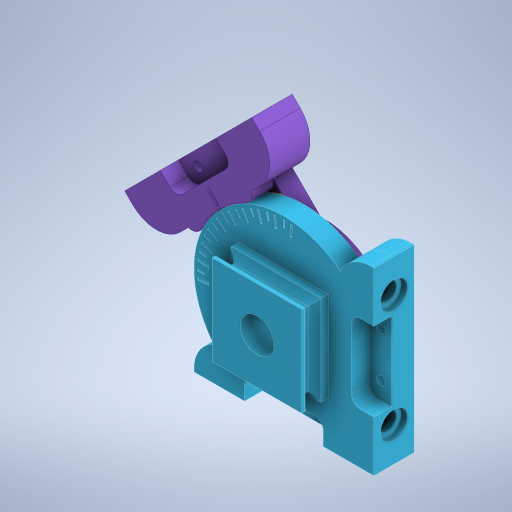
# Autodesk Inventor part: Rail-AdjustableAngle
Saved by Autodesk Inventor 2023.1 (Build 271208000, 208)
## iProperties
Created: 2023-06-07
Part Number: Rail-AdjustableAngle
Material: ABS Plastic
Document SubType Name: Modeling
Designer: hello
Density: 1.06 g/cm^3
Appearance: Turquoise
Author: hello
Autodesk Inventor part; units mm, degrees
ref_plane "YZ Plane" through (0, 0, 0) normal (1, 0, 0) x (0, 1, 0)
ref_plane "XZ Plane" through (0, 0, 0) normal (0, 1, 0) x (-1, 0, 0)
ref_plane "XY Plane" through (0, 0, 0) normal (0, 0, 1) x (1, 0, 0)
sketch "Sketch1" plane through (0, 0, 0) normal (0, 0, 1) x (1, 0, 0)
  line L0 (-40, 40) -> (40, 40)
  line L1 (40, 40) -> (40, -40)
  line L2 (40, -40) -> (-40, -40)
  line L3 (-40, -40) -> (-40, 40)
  line L4 (-40, 40) -> (40, -40) construction
  line L5 (40, 40) -> (-40, -40) construction
  line L6 (40, 0) -> (-40, 0) construction
  arc A0 (0, 40) -> (-39.8798, -3.0986) centre (0, 0) ccw
  point P0 (0, 0)
  point P1 (-40, -18.9335)
  point P2 (0, 0)
  point P3 (-40, 0)
  dimension "d0" = 80
  dimension "d1" = 80
  constraints: 14 end point, 6 midpoint, 2 horizontal, 2 parallel, 2 point on circle, 1 centre point, 1 coincident, 1 perpendicular, 1 point on line
  measures "d0" distance of L1.end L2.end
  measures "d1" distance of L0.end L1.end
extrude "Extrusion1" add sketch "Sketch1" along normal blind 18 contours L0 L1 L2 L3 A0
sketch "Sketch2" plane through (40, -40, 0) normal (1, 0, 0) x (0, 0, -1)
  line L0 (0, 0) -> (0, 80) projected
  line L1 (0, 80) -> (-18, 80) projected
  line L2 (-18, 0) -> (-18, 80) projected
  line L3 (0, 0) -> (-18, 0) projected
  line L4 (-9, 15) -> (-9, 65)
  point P0 (0, 40)
  point P1 (-9, 40)
  point P2 (0, 40)
  point P3 (-9, 0)
  dimension "d7" = 50
  constraints: 3 midpoint, 2 coincident, 2 end point, 1 horizontal alignment, 1 vertical, 1 vertical alignment
  measures "d7" distance of L4.start L4.end
hole "Hole1" at (40, -25, 9) at (40, 25, 9) direction (-1, 0, 0) diameter 8.05 depth 15 counterbore diameter 12 counterbore depth 3
sketch "Sketch3" plane through (-40, -40, 0) normal (0, -1, 0) x (1, 0, 0)
  line L0 (0, 0) -> (80, 0) projected
  line L1 (80, 0) -> (80, 18) projected
  line L2 (0, 18) -> (80, 18) projected
  line L3 (0, 0) -> (0, 18) projected
  line L4 (15, 9) -> (65, 9)
  point P0 (40, 0)
  point P1 (40, 9)
  point P2 (0, 9)
  point P3 (40, 0)
  dimension "d15" = 50
  constraints: 3 midpoint, 2 coincident, 2 end point, 1 horizontal, 1 horizontal alignment, 1 vertical alignment
  measures "d15" distance of L4.start L4.end
hole "Hole2" at (-25, -40, 9) at (25, -40, 9) direction (0, 1, 0) diameter 8.05 depth 15 counterbore diameter 12 counterbore depth 3
sketch "Sketch4" plane through (0, 0, 18) normal (0, 0, 1) x (1, 0, 0)
  line L0 (40, -40) -> (40, 40) projected
  line L1 (34, -17.5) -> (40, -17.5)
  line L2 (40, -17.5) -> (40, 17.5)
  line L3 (40, 17.5) -> (34, 17.5)
  line L4 (30, 13.5) -> (30, -13.5)
  arc A0 (30, -13.5) -> (34, -17.5) centre (34, -13.5) ccw
  arc A1 (34, 17.5) -> (30, 13.5) centre (34, 13.5) ccw
  point P0 (0, 0)
  point P1 (30, -17.5)
  point P2 (30, 17.5)
  point P3 (40, 0)
  dimension "d23" = 35
  dimension "d24" = 10
  dimension "d25" = 4
  constraints: 8 end point, 4 point on circle, 4 point on line, 4 tangent, 2 centre point, 2 midpoint, 2 parallel, 1 equal radius, 1 horizontal, 1 perpendicular
  measures "d23" distance of point (30, 17.5) point (30, -17.5)
  measures "d24" distance of point (30, -17.5) L1.end
  measures "d25" radius of A0
extrude "Extrusion2" cut sketch "Sketch4" against normal blind 8
sketch "Sketch5" plane through (0, 0, 10) normal (0, 0, 1) x (1, 0, 0)
  line L0 (35, -10) -> (35, 10)
  line L1 (40, 17.5) -> (40, -17.5) projected
  point P0 (0, 0)
  point P1 (35, 0)
  point P2 (40, 0)
  dimension "d28" = 20
  dimension "d29" = 5
  constraints: 2 coincident, 2 end point, 2 midpoint, 1 horizontal alignment, 1 vertical
  measures "d28" distance of L0.start L0.end
  measures "d29" distance between parallel lines of L1 L0
hole "Hole3" at (35, -10, 10) at (35, 10, 10) direction (0, 0, -1) diameter 4 depth 5
pattern_circular "Circular Pattern1" count 2 over 90 about axis through (0, 0, -10) along (0, 0, -1) of "Extrusion2", "Hole3"
sketch "Sketch6" plane through (0, 0, 18) normal (0, 0, 1) x (1, 0, 0)
  line L0 (-20, 20) -> (20, 20)
  line L1 (20, 20) -> (20, -20)
  line L2 (20, -20) -> (-20, -20)
  line L3 (-20, -20) -> (-20, 20)
  line L4 (-20, 20) -> (20, -20) construction
  line L5 (20, 20) -> (-20, -20) construction
  point P0 (0, 0)
  dimension "d40" = 40
  dimension "d41" = 40
  constraints: 12 end point, 2 midpoint, 2 parallel, 1 horizontal, 1 perpendicular
  measures "d40" distance of L1.end L2.end
  measures "d41" distance of L0.end L1.end
extrude "Extrusion3" add sketch "Sketch6" along normal blind 12
sketch "Sketch11" plane through (-20, -20, 18) normal (0, -1, 0) x (1, 0, 0)
  line L0 (40, 0) -> (0, 0) projected
  line L1 (40, 0) -> (40, 12) projected
  line L2 (0, 12) -> (40, 12) construction
  line L3 (0, 0) -> (0, 12) construction
  line L4 (0, 12) -> (40, 12) projected
  line L5 (0, 12) -> (0, 10)
  line L6 (0, 0) -> (0, 12) projected
  circle A0 centre (0, 6.7947) radius 3 construction
  arc A1 (4.3, 6.7947) -> (0, 10) centre (-2.036, 2.7817) ccw
  arc A2 (0, 3.5894) -> (4.3, 6.7947) centre (-2.036, 10.8077) ccw
  line L7 (3.5, 7.8415) -> (3.5, 5.7479)
  line L8 (0, 10) -> (0, 3.5894)
  point P0 (20, -18)
  point P1 (0, 11)
  dimension "d65" = 2
  dimension "d66" = 6
  dimension "d67" = 7.5
  dimension "d68" = 7.5
  dimension "d69" = 3.5
  dimension "d70" = 4.3
  constraints: 6 end point, 6 point on circle, 3 centre point, 3 point on line, 2 tangent, 2 vertical, 1 horizontal alignment, 1 midpoint
  measures "d65" distance of L2.start L5.end
  measures "d66" diameter of A0
  measures "d67" radius of A1
  measures "d68" radius of A2
  measures "d69" distance from line of L7 point (0, 11)
  measures "d70" distance from line of A1.start L3
extrude "Extrusion5" cut sketch "Sketch11" against normal through all contours L6 A1 L7 A2
pattern_circular "Circular Pattern2" count 4 over 360 about axis through (0, 0, -10) along (0, 0, 1) of "Extrusion5"
fillet "Fillet1" radius 1.5 4 edges at (0, -20, 28) (-20, 0, 28) (0, 20, 28) (20, 0, 28)
sketch "Sketch12" plane through (0, 0, 30) normal (0, 0, 1) x (1, 0, 0)
  point P0 (0, 0)
  point P1 (0, 0)
  constraints: 1 coincident
hole "Hole6" at (0, 0, 30) direction (0, 0, -1) diameter 5.5 end through all counterbore diameter 15 counterbore depth 20 clearance for "Hex Head Cap Screw ISO 24017" size "M5" standard "ISO"
sketch "Sketch17" plane through (0, 0, 0) normal (0, 0, -1) x (-1, 0, 0)
  arc A0 (40, 0) -> (0, 40) centre (0, 0) ccw projected
  arc A1 (31.225, -25) -> (40, 0) centre (0, 0) ccw
  line L0 (40, 0) -> (40, -40) projected
  line L1 (40, 0) -> (40, -25)
  line L2 (31.225, -25) -> (40, -25)
  line L3 (-40, 40) -> (0, 40) projected
  arc A2 (0, 40) -> (-25, 31.225) centre (0, 0) ccw
  line L4 (-25, 31.225) -> (-25, 40)
  line L5 (-25, 40) -> (0, 40)
  point P0 (0, 0)
  dimension "d118" = 40
  dimension "d119" = 25
  dimension "d122" = 40
  dimension "d123" = 25
  constraints: 8 end point, 4 point on circle, 3 perpendicular, 3 tangent, 2 centre point, 2 point on line
  measures "d118" radius of A1
  measures "d119" vertical distance of L2.start point (0, 0)
  measures "d122" radius of A2
  measures "d123" horizontal distance of point (0, 0) L4.start
extrude "Extrusion8" cut sketch "Sketch17" against normal through all
sketch "Sketch18" plane through (0, 0, 0) normal (0, 0, -1) x (-1, 0, 0)
  arc A0 (31.225, -25) -> (-25, 31.225) centre (0, 0) ccw projected
  arc A1 (31.225, -25) -> (-25, 31.225) centre (0, 0) ccw projected
  line L0 (-25, 31.225) -> (31.225, -25)
  circle A2 centre (0, 0) radius 2.75 projected
  circle A3 centre (0, 0) radius 30
  point P0 (24.0961, -17.8711)
  point P1 (-17.8711, 24.0961)
  dimension "d124" = 60
  constraints: 2 end point, 1 centre point, 1 coincident
  measures "d124" diameter of A3
extrude "Extrusion9" cut sketch "Sketch18" against normal blind 9
sketch "Sketch19" plane through (0, 0, 0) normal (0, 1, 0) x (-1, 0, 0)
  line L0 (-2.75, 9) -> (2.75, 9) projected
  line L1 (2.75, 9) -> (2.75, 0)
  line L2 (2.75, 9) -> (25, 9)
  line L3 (24.0961, 9) -> (-30, 9) projected
  line L4 (25, 9) -> (25, 0)
  line L5 (40, 0) -> (-40, 0) projected
  line L6 (2.75, 0) -> (25, 0)
  line L7 (0, 0) -> (0, 9)
  circle A0 centre (25, 4.5) radius 3
  point P0 (-17.8711, 9)
  point P1 (25, 1.5)
  point P2 (25, 7.5)
  dimension "d128" = 50
  dimension "d129" = 6
  constraints: 10 end point, 3 point on line, 2 perpendicular, 1 centre point, 1 collinear, 1 midpoint, 1 vertical
  measures "d128" diameter of L4 L7
  measures "d129" diameter of A0
revolve "Revolution1" add sketch "Sketch19" angle 360 about axis through (0, 0, 0) along (0, 0, 1) contours L2 L4 A0 L5 L1
fillet "Fillet3" radius 15 2 edges at (17.8711, 24.0961, 4.5) (-24.0961, -17.8711, 4.5)
fillet "Fillet4" radius 15 2 edges at (25, 40, 9) (-40, -25, 9)
sketch "Sketch20" plane through (0, 0, 0) normal (0, 1, 0) x (-1, 0, 0)
  arc A0 (25, 7.5) -> (25, 1.5) centre (25, 4.5) ccw projected
  line L0 (25, 7.5) -> (25, 9) projected
  line L1 (25, 0) -> (25, 1.5) projected
  arc A1 (25.1, 7.2982) -> (25.1, 1.7018) centre (25, 4.5) ccw
  line L2 (25.1, 7.2982) -> (25.1, 9)
  line L3 (25.1, 0) -> (25.1, 1.7018)
  line L4 (25.1, 0) -> (29.9, 0)
  line L5 (40, 0) -> (-40, 0) projected
  line L6 (29.9, 0) -> (29.9, 8.6)
  line L7 (29.9, 8.6) -> (25.1, 8.6)
  line L8 (0, -6) -> (0, 36) projected
  point P0 (0, 0)
  dimension "d133" = 0.2
  dimension "d134" = 0.1
  dimension "d135" = 0.1
  dimension "d136" = 0.4
  dimension "d137" = 4.9
  constraints: 10 end point, 2 parallel, 2 point on circle, 2 point on line, 1 centre point, 1 horizontal, 1 horizontal alignment, 1 vertical
  measures "d133" radial gap between concentric circles of A0 A1
  measures "d134" distance between parallel lines of L0 L2
  measures "d135" distance between parallel lines of L1 L3
  measures "d136" distance from line of L2.end L7
  measures "d137" distance from line of L6 A0.centre
revolve "Revolution2" add sketch "Sketch20" angle 360 about axis through (0, 0, -10) along (0, 0, 1) separate body
sketch "Sketch21" plane through (0, 0, 0) normal (0, 0, -1) x (-1, 0, 0)
  circle A0 centre (0, 0) radius 29.9 projected
  circle A1 centre (0, 0) radius 29.9 projected
  line L0 (1.5743, 29.8585) -> (14.3022, 42.5865)
  line L1 (14.3022, 42.5865) -> (42.5865, 14.3022)
  line L2 (42.5865, 14.3022) -> (29.8585, 1.5743)
  circle A2 centre (0, 0) radius 2.75 projected
  line L3 (0, 0) -> (28.4443, 28.4443)
  line L4 (0, 0) -> (0, 11.9435)
  line L5 (14.3022, 42.5865) -> (0.16, 56.7286)
  line L6 (0.16, 56.7286) -> (14.3022, 70.8707)
  line L7 (14.3022, 70.8707) -> (70.8707, 14.3022)
  line L8 (70.8707, 14.3022) -> (56.7286, 0.16)
  line L9 (56.7286, 0.16) -> (42.5865, 14.3022)
  point P0 (29.8585, 1.5743)
  dimension "d139" = 40
  dimension "d140" = 18
  dimension "d141" = 45
  dimension "d142" = 20
  dimension "d143" = 80
  constraints: 20 end point, 7 perpendicular, 2 collinear, 2 point on circle, 1 midpoint, 1 vertical
  measures "d139" distance of L0.end L1.end
  measures "d140" distance of L1.end L2.end
  measures "d141" angle of L3 L4
  measures "d142" distance of L7.end L8.end
  measures "d143" distance of L6.end L7.end
extrude "Extrusion10" add sketch "Sketch21" against normal up to surface (8.6 mm away) contours A0 L3 L1 L2 | L0 L1 L3 A0 | L1 L5 L6 L7 L8 L9 bodies 2
sketch "Sketch22" plane through (0, 0, 8.6) normal (0, 0, 1) x (0.7071068, -0.7071068, 0)
  circle A0 centre (0, 0) radius 25.1 projected
  arc A1 (-22.2263, -20) -> (-22.2263, 20) centre (0, 0) ccw projected
  line L0 (-40.2263, 20) -> (-22.2263, 20) projected
  line L1 (-40.2263, 40) -> (-40.2263, 20) projected
  line L2 (-60.2263, 40) -> (-40.2263, 40) projected
  line L3 (-60.2263, -40) -> (-60.2263, 40) projected
  line L4 (-40.2263, -40) -> (-60.2263, -40) projected
  line L5 (-40.2263, -20) -> (-40.2263, -40) projected
  line L6 (-22.2263, -20) -> (-40.2263, -20) projected
  circle A2 centre (0, 0) radius 2.75 projected
  circle A3 centre (0, 0) radius 40.25
  point P0 (-34.9294, -20)
  point P1 (-34.9294, 20)
  dimension "d146" = 80.5
  constraints: 1 centre point, 1 coincident
  measures "d146" diameter of A3
extrude "Extrusion11" add sketch "Sketch22" along normal up to surface (9.4 mm away) contours L6 L5 L4 L3 L2 L1 L0 A3 bodies 2
sketch "Sketch23" plane through (-14.3022, 70.8707, 0) normal (-0.7071068, 0.7071068, 0) x (-0.7071068, -0.7071068, 0)
  line L0 (0, 0) -> (0, 18) projected
  line L1 (80, 0) -> (0, 0) projected
  line L2 (80, 0) -> (80, 18) projected
  line L3 (80, 18) -> (0, 18) projected
  line L4 (15, 9) -> (65, 9)
  line L5 (80, 0) -> (0, 0) projected
  point P0 (40, 0)
  point P1 (40, 9)
  point P2 (0, 9)
  point P3 (40, 0)
  dimension "d149" = 50
  constraints: 3 midpoint, 2 coincident, 2 end point, 1 horizontal, 1 horizontal alignment, 1 vertical alignment
  measures "d149" distance of L4.start L4.end
hole "Hole7" at (-24.9088, 60.2641, 9) at (-60.2641, 24.9088, 9) direction (0.7071068, -0.7071068, 0) diameter 8.05 depth 15 counterbore diameter 12 counterbore depth 3 bodies 2
fillet "Fillet5" radius 5 2 edges at (-10.5567, 38.8409, 13.3) (-38.8409, 10.5567, 13.3)
sketch "Sketch24" plane through (0, 0, 0) normal (0, 1, 0) x (-1, 0, 0)
  line L0 (36.5062, 8.6) -> (16.9516, 8.6) construction
  line L1 (40, 9) -> (-25, 9) construction
  line L2 (25, 7.5) -> (25, 9) construction
  line L3 (29.9, 8.6) -> (-29.9, 8.6) construction
  line L4 (25, 9) -> (29.9, 9)
  line L5 (29.9, 9) -> (29.9, 8.6)
  line L6 (29.9, 8.6) -> (25, 8.6)
  line L7 (25, 8.6) -> (25, 9)
  line L8 (0, -6) -> (0, 36) projected
  point P0 (0, 0)
  point P1 (31.225, 9)
  point P2 (29.8585, 8.6)
  point P3 (1.5743, 8.6)
  constraints: 8 end point, 2 parallel, 1 horizontal, 1 perpendicular
revolve "Revolution3" add sketch "Sketch24" angle 360 about axis through (0, 0, -10) along (0, 0, 1) separate body
sketch "Sketch25" plane through (0, 0, 9) normal (0, 0, -1) x (-1, 0, 0)
  circle A0 centre (0, 0) radius 25.1 projected
  line L0 (29.8585, 1.5743) -> (42.5865, 14.3022) projected
  line L1 (14.3022, 42.5865) -> (1.5743, 29.8585) projected
  arc A1 (31.225, -25) -> (-25, 31.225) centre (0, 0) ccw projected
  arc A2 (31.225, -25) -> (-25, 31.225) centre (0, 0) ccw projected
  line L2 (29.8585, 1.5743) -> (24.8662, -3.4181)
  line L3 (1.5743, 29.8585) -> (-3.4181, 24.8662)
  point P0 (38.637, 10.3528)
  point P1 (10.3528, 38.637)
  constraints: 4 end point, 2 point on circle, 1 collinear, 1 parallel
extrude "Extrusion12" add sketch "Sketch25" along normal up to surface (0.4 mm away) contours A0 L3 L1 A1 L0 L2 bodies 3
sketch "Sketch26" plane through (-70.8707, 14.3022, 18) normal (0, 0, 1) x (0.7071068, -0.7071068, 0)
  line L0 (0, 0) -> (0, 80) projected
  line L1 (6, 57.5) -> (0, 57.5)
  line L2 (0, 57.5) -> (0, 22.5)
  line L3 (0, 22.5) -> (6, 22.5)
  line L4 (10, 26.5) -> (10, 53.5)
  arc A0 (10, 53.5) -> (6, 57.5) centre (6, 53.5) ccw
  arc A1 (6, 22.5) -> (10, 26.5) centre (6, 26.5) ccw
  point P0 (60.2263, 40)
  point P1 (10, 22.5)
  point P2 (0, 40)
  point P3 (0, 57.5)
  point P4 (0, 22.5)
  dimension "d161" = 10
  dimension "d162" = 35
  dimension "d163" = 4
  constraints: 8 end point, 4 point on circle, 4 tangent, 2 centre point, 2 midpoint, 2 parallel, 2 point on line, 1 equal radius, 1 horizontal, 1 perpendicular
  measures "d161" distance of point (10, 22.5) L2.end
  measures "d162" distance of L2.end L1.end
  measures "d163" radius of A0
extrude "Extrusion13" cut sketch "Sketch26" against normal blind 8 bodies 2
sketch "Sketch27" plane through (-70.8707, 14.3022, 10) normal (0, 0, 1) x (0.7071068, 0.7071068, 0)
  line L0 (57.5, 0) -> (57.5, -6) projected
  line L1 (22.5, 0) -> (57.5, 0) projected
  line L2 (22.5, -6) -> (22.5, 0) projected
  arc A0 (22.5, -6) -> (26.5, -10) centre (26.5, -6) ccw projected
  line L3 (53.5, -10) -> (26.5, -10) projected
  arc A1 (53.5, -10) -> (57.5, -6) centre (53.5, -6) ccw projected
  line L4 (50, -5) -> (30, -5)
  line L5 (22.5, 0) -> (57.5, 0) projected
  line L6 (40, 0) -> (40, -10)
  point P0 (40, -60.2263)
  point P1 (40, -5)
  dimension "d166" = 20
  constraints: 4 end point, 4 midpoint, 2 coincident, 1 horizontal
  measures "d166" distance of L4.start L4.end
hole "Hole8" at (-31.9798, 46.122, 10) at (-46.122, 31.9798, 10) direction (0, 0, -1) diameter 4 depth 5 bodies 2
fillet "Fillet6" radius 15 2 edges at (-0.16, 56.7286, 9) (-56.7286, 0.16, 9)
sketch "Sketch29" plane through (0, 0, 18) normal (0, 0, 1) x (1, 0, 0)
  line L0 (-25.3851, 24.8194) -> (-27.5065, 26.9408)
  line L1 (-27.5065, 26.9408) -> (-26.9408, 27.5065)
  line L2 (-26.9408, 27.5065) -> (-24.8194, 25.3851)
  line L3 (-24.8194, 25.3851) -> (-25.3851, 24.8194)
  line L4 (-25.3851, 24.8194) -> (-26.9408, 27.5065) construction
  line L5 (-27.5065, 26.9408) -> (-24.8194, 25.3851) construction
  circle A0 centre (0, 0) radius 2.75 projected
  line L6 (0, 0) -> (-26.163, 26.163)
  line L7 (0, 0) -> (0, 5.2845)
  line L8 (-21.0569, 32.2338) -> (-19.3902, 29.7394)
  line L9 (-19.3902, 29.7394) -> (-20.0553, 29.2949)
  line L10 (-20.0553, 29.2949) -> (-21.722, 31.7894)
  line L11 (-21.722, 31.7894) -> (-21.0569, 32.2338)
  line L12 (-14.3638, 35.7224) -> (-13.2157, 32.9508)
  line L13 (-13.2157, 32.9508) -> (-13.9548, 32.6447)
  line L14 (-13.9548, 32.6447) -> (-15.1029, 35.4163)
  line L15 (-15.1029, 35.4163) -> (-14.3638, 35.7224)
  line L16 (-7.1187, 37.8383) -> (-6.5334, 34.8959)
  line L17 (-6.5334, 34.8959) -> (-7.318, 34.7398)
  line L18 (-7.318, 34.7398) -> (-7.9033, 37.6822)
  line L19 (-7.9033, 37.6822) -> (-7.1187, 37.8383)
  line L20 (0.4, 38.5) -> (0.4, 35.5)
  line L21 (0.4, 35.5) -> (-0.4, 35.5)
  line L22 (-0.4, 35.5) -> (-0.4, 38.5)
  line L23 (-0.4, 38.5) -> (0.4, 38.5)
  line L24 (-31.7894, 21.722) -> (-29.2949, 20.0553)
  line L25 (-29.2949, 20.0553) -> (-29.7394, 19.3902)
  line L26 (-29.7394, 19.3902) -> (-32.2338, 21.0569)
  line L27 (-32.2338, 21.0569) -> (-31.7894, 21.722)
  line L28 (-35.4163, 15.1029) -> (-32.6447, 13.9548)
  line L29 (-32.6447, 13.9548) -> (-32.9508, 13.2157)
  line L30 (-32.9508, 13.2157) -> (-35.7224, 14.3638)
  line L31 (-35.7224, 14.3638) -> (-35.4163, 15.1029)
  line L32 (-37.6822, 7.9033) -> (-34.7398, 7.318)
  line L33 (-34.7398, 7.318) -> (-34.8959, 6.5334)
  line L34 (-34.8959, 6.5334) -> (-37.8383, 7.1187)
  line L35 (-37.8383, 7.1187) -> (-37.6822, 7.9033)
  line L36 (-38.5, 0.4) -> (-35.5, 0.4)
  line L37 (-35.5, 0.4) -> (-35.5, -0.4)
  line L38 (-35.5, -0.4) -> (-38.5, -0.4)
  line L39 (-38.5, -0.4) -> (-38.5, 0.4)
  line L40 (-21.1504, 25.9839) -> (-24.3643, 29.8141)
  line L41 (-24.3643, 29.8141) -> (-25.1303, 29.1713)
  line L42 (-25.1303, 29.1713) -> (-21.9164, 25.3411)
  line L43 (-21.9164, 25.3411) -> (-21.1504, 25.9839)
  line L44 (-21.1504, 25.9839) -> (-25.1303, 29.1713) construction
  line L45 (-24.3643, 29.8141) -> (-21.9164, 25.3411) construction
  circle A1 centre (0, 0) radius 2.75 projected
  line L46 (0, 0) -> (-23.1404, 27.5776)
  line L47 (-27.5065, 26.9408) -> (-27.7135, 27.7135)
  line L48 (-27.7135, 27.7135) -> (-26.9408, 27.5065)
  line L49 (-18.0797, 33.9945) -> (-18.9564, 33.5135)
  line L50 (-18.9564, 33.5135) -> (-16.5515, 29.1299)
  line L51 (-15.6748, 29.6108) -> (-18.0797, 33.9945)
  line L52 (-16.5515, 29.1299) -> (-15.6748, 29.6108)
  line L53 (-11.1003, 36.8685) -> (-12.054, 36.5677)
  line L54 (-12.054, 36.5677) -> (-10.5505, 31.7992)
  line L55 (-9.5968, 32.0999) -> (-11.1003, 36.8685)
  line L56 (-10.5505, 31.7992) -> (-9.5968, 32.0999)
  line L57 (-3.6943, 38.3256) -> (-4.6884, 38.2167)
  line L58 (-4.6884, 38.2167) -> (-4.1441, 33.2465)
  line L59 (-3.15, 33.3553) -> (-3.6943, 38.3256)
  line L60 (-4.1441, 33.2465) -> (-3.15, 33.3553)
  line L61 (-29.6055, 24.6174) -> (-30.2348, 23.8403)
  line L62 (-30.2348, 23.8403) -> (-26.349, 20.6937)
  line L63 (-25.7197, 21.4708) -> (-29.6055, 24.6174)
  line L64 (-26.349, 20.6937) -> (-25.7197, 21.4708)
  line L65 (-33.7587, 18.5161) -> (-34.2282, 17.6332)
  line L66 (-34.2282, 17.6332) -> (-29.8135, 15.2858)
  line L67 (-29.344, 16.1688) -> (-33.7587, 18.5161)
  line L68 (-29.8135, 15.2858) -> (-29.344, 16.1688)
  line L69 (-36.6715, 11.7345) -> (-36.9639, 10.7782)
  line L70 (-36.9639, 10.7782) -> (-32.1824, 9.3163)
  line L71 (-31.89, 10.2726) -> (-36.6715, 11.7345)
  line L72 (-32.1824, 9.3163) -> (-31.89, 10.2726)
  line L73 (-38.2368, 4.5216) -> (-38.3414, 3.5271)
  line L74 (-38.3414, 3.5271) -> (-33.3687, 3.0044)
  line L75 (-33.2642, 3.999) -> (-38.2368, 4.5216)
  line L76 (-33.3687, 3.0044) -> (-33.2642, 3.999)
  line L77 (-38.3971, -2.8574) -> (-38.3099, -3.8536)
  line L78 (-38.3099, -3.8536) -> (-33.3289, -3.4178)
  line L79 (-33.4161, -2.4216) -> (-38.3971, -2.8574)
  line L80 (-33.3289, -3.4178) -> (-33.4161, -2.4216)
  line L81 (3.8536, 38.3099) -> (2.8574, 38.3971)
  line L82 (2.8574, 38.3971) -> (2.4216, 33.4161)
  line L83 (3.4178, 33.3289) -> (3.8536, 38.3099)
  line L84 (2.4216, 33.4161) -> (3.4178, 33.3289)
  point P0 (-25.1023, 25.1023)
  point P1 (-19.7227, 29.5172)
  point P2 (-13.5853, 32.7977)
  point P3 (-6.9257, 34.8179)
  point P4 (0, 35.5)
  point P5 (-29.5172, 19.7227)
  point P6 (-32.7977, 13.5853)
  point P7 (-34.8179, 6.9257)
  point P8 (-35.5, 0)
  point P9 (-21.5334, 25.6625)
  point P10 (-16.1131, 29.3703)
  point P11 (-10.0736, 31.9495)
  point P12 (-3.647, 33.3009)
  point P13 (-26.0344, 21.0822)
  point P14 (-29.5787, 15.7273)
  point P15 (-32.0362, 9.7945)
  point P16 (-33.3165, 3.5017)
  point P17 (-33.3725, -2.9197)
  point P18 (2.9197, 33.3725)
  dimension "d175" = 0.8
  dimension "d176" = 45
  dimension "d177" = 3
  dimension "d178" = 37
  dimension "d182" = 45
  dimension "d186" = 45
  dimension "d190" = 1
  dimension "d191" = 5
  dimension "d192" = 40
  dimension "d193" = 36
  dimension "d195" = 0.8
  dimension "d198" = 45
  dimension "d202" = 55
  constraints: 170 end point, 6 midpoint, 4 parallel, 2 perpendicular, 2 point on line, 1 equal length, 1 vertical, 157 other
  measures "d175" distance of L0.end L1.end
  measures "d176" angle of L6 L7
  measures "d177" distance of L0.start L0.end
  measures "d178" distance of L6.start L6.end
  measures "d190" distance of L40.end L41.end
  measures "d191" distance of L41.end L42.end
  measures "d192" angle of L46 L7
  measures "d193" distance of L46.start L46.end
  measures "d195" distance of L0.end L47.end
extrude "Extrusion14" cut sketch "Sketch29" against normal blind 0.5 contours L0 L1 L2 L3 | L47 L48 L1 | L8 L9 L10 L11 | L12 L13 L14 L15 | L16 L17 L18 L19 | L20 L21 L22 L23 | L24 L25 L26 L27 | L28 L29 L30 L31 | L32 L33 L34 L35 | L36 L37 L38 L39 | L43 L42 L41 L40 | L51 L52 L50 L49 | L55 L56 L54 L53 | L59 L60 L58 L57 | L63 L64 L62 L61 | L67 L68 L66 L65 | L71 L72 L70 L69 | L75 L76 L74 L73 | L79 L80 L78 L77 | L83 L84 L82 L81 bodies 1
sketch "Sketch30" plane through (-47.8898, 28.7979, 18) normal (0, 0, 1) x (1, 0, 0)
  arc A0 (-19.4454, -18.0312) -> (1.7678, -18.0312) centre (-8.8388, -7.4246) ccw projected
  line L0 (5.3033, -14.4957) -> (1.7678, -18.0312) projected
  arc A1 (5.3033, -14.4957) -> (11.3835, -11.8463) centre (6.8486, -9.7405) ccw projected
  arc A2 (30.9381, 7.7084) -> (11.3835, -11.8463) centre (47.8898, -28.7979) ccw projected
  arc A3 (30.9381, 7.7084) -> (33.5876, 13.7886) centre (28.8324, 12.2433) ccw projected
  line L1 (37.1231, 17.3241) -> (33.5876, 13.7886) projected
  arc A4 (37.1231, 17.3241) -> (37.1231, 38.5373) centre (26.5165, 27.9307) ccw projected
  line L2 (33.5876, 42.0729) -> (37.1231, 38.5373) projected
  line L3 (17.6777, 26.163) -> (33.5876, 42.0729) projected
  line L4 (17.6777, 26.163) -> (21.9203, 21.9203) projected
  arc A5 (21.9203, 16.2635) -> (21.9203, 21.9203) centre (19.0919, 19.0919) ccw projected
  line L5 (21.9203, 16.2635) -> (2.8284, -2.8284) projected
  arc A6 (-2.8284, -2.8284) -> (2.8284, -2.8284) centre (0, 0) ccw projected
  line L6 (-2.8284, -2.8284) -> (-7.0711, 1.4142) projected
  line L7 (-22.981, -14.4957) -> (-7.0711, 1.4142) projected
  line L8 (-19.4454, -18.0312) -> (-22.981, -14.4957) projected
  line L9 (20.1762, -1.0844) -> (20.949, -1.2914) projected
  line L10 (20.1762, -1.0844) -> (12.3744, 6.7175) construction
  line L11 (21.9203, 16.2635) -> (2.8284, -2.8284) projected
  line L12 (13.6237, 4.7611) -> (18.2198, 0.1649)
  line L13 (18.2198, 0.1649) -> (18.927, 0.872)
  line L14 (18.927, 0.872) -> (14.3308, 5.4682)
  line L15 (14.3308, 5.4682) -> (13.6237, 4.7611)
  line L16 (13.6237, 4.7611) -> (18.927, 0.872) construction
  line L17 (18.2198, 0.1649) -> (14.3308, 5.4682) construction
  line L18 (18.2198, 0.1649) -> (19.1858, -0.0939)
  line L19 (19.1858, -0.0939) -> (18.927, 0.872)
  point P0 (16.2753, 2.8166)
  dimension "d204" = 1
  dimension "d205" = 6.5
  constraints: 18 end point, 4 midpoint, 2 equal length, 2 parallel, 1 perpendicular, 1 point on line
  measures "d204" distance of L13.end L12.end
  measures "d205" distance of L12.start L12.end
extrude "Extrusion15" cut sketch "Sketch30" against normal blind 0.5 contours L15 L14 L13 L12 | L13 L19 L18 bodies 2
equation "\"d122\" = d118"
equation "\"d123\" = d119"
body "Solid1"
body "Solid2"
